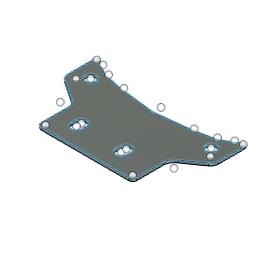
prop bracket (Autodesk Fusion 360 design; units mm, degrees)
Autodesk Fusion 360 part; units mm, degrees
sketch "sketch 344" plane through (0, 0, 1390) normal (0, 0, -1) x (1, 0, 0)
  circle A0 centre (6470.3364, 391.9726) radius 6.75
  circle A1 centre (6317.9364, 391.9726) radius 6.75
  line L0 (6410.85, 446.765) -> (6410.85, 453.115)
  arc A2 (6410.85, 453.115) -> (6424.35, 453.115) centre (6417.6, 453.115) cw
  line L1 (6424.35, 453.115) -> (6424.35, 446.765)
  arc A3 (6424.35, 446.765) -> (6410.85, 446.765) centre (6417.6, 446.765) cw
  line L2 (6367.75, 453.172) -> (6367.75, 446.828)
  arc A4 (6367.75, 446.828) -> (6354.25, 446.828) centre (6361, 446.828) cw
  line L3 (6354.25, 446.828) -> (6354.25, 453.172)
  arc A5 (6354.25, 453.172) -> (6367.75, 453.172) centre (6361, 453.172) cw
  line L4 (6455.7, 437.7) -> (6455.7, 471.6807)
  arc A6 (6455.7, 471.6807) -> (6450.62, 476.7607) centre (6450.62, 471.6807) ccw
  line L5 (6340.255, 476.7607) -> (6450.62, 476.7607)
  arc A7 (6340.255, 476.7607) -> (6335.175, 471.6807) centre (6340.255, 471.6807) ccw
  line L6 (6335.175, 437.7001) -> (6335.175, 471.6807)
  arc A8 (6330.4473, 428.3006) -> (6335.175, 437.7001) centre (6324.513, 437.1741) ccw
  line L7 (6303.3983, 410.211) -> (6330.4473, 428.3006)
  arc A9 (6303.3983, 410.211) -> (6298.8864, 401.7656) centre (6309.0464, 401.7656) ccw
  line L8 (6298.8864, 401.7656) -> (6298.8864, 367.9042)
  arc A10 (6298.8864, 367.9042) -> (6303.0986, 365.9924) centre (6301.4264, 367.9042) ccw
  line L9 (6309.1204, 371.2594) -> (6303.0986, 365.9924)
  arc A11 (6309.6287, 371.6052) -> (6309.1204, 371.2594) centre (6310.7926, 369.3475) ccw
  line L10 (6323.9162, 378.9712) -> (6309.6287, 371.6052)
  arc A12 (6324.5666, 379.2011) -> (6323.9162, 378.9712) centre (6325.0801, 376.7135) ccw
  line L11 (6349.1728, 384.2811) -> (6324.5666, 379.2011)
  arc A13 (6349.398, 384.3171) -> (6349.1728, 384.2811) centre (6349.6864, 381.7935) ccw
  line L12 (6349.398, 384.3171) -> (6392.9828, 389.2982)
  arc A14 (6395.29, 389.2982) -> (6392.9828, 389.2982) centre (6394.1364, 379.2039) ccw
  line L13 (6395.29, 389.2982) -> (6438.8748, 384.3171)
  arc A15 (6439.0999, 384.2811) -> (6438.8748, 384.3171) centre (6438.5864, 381.7935) ccw
  line L14 (6439.0999, 384.2811) -> (6463.7062, 379.2011)
  arc A16 (6464.3565, 378.9712) -> (6463.7062, 379.2011) centre (6463.1926, 376.7135) ccw
  line L15 (6464.3565, 378.9712) -> (6478.644, 371.6054)
  arc A17 (6479.1524, 371.2596) -> (6478.644, 371.6054) centre (6477.4801, 369.3477) ccw
  line L16 (6479.1524, 371.2596) -> (6485.1741, 365.9925)
  arc A18 (6485.1741, 365.9925) -> (6489.3864, 367.9043) centre (6486.8464, 367.9043) ccw
  line L17 (6489.3864, 401.9194) -> (6489.3864, 367.9043)
  arc A19 (6489.3864, 401.9194) -> (6485.0731, 410.2286) centre (6479.2264, 401.9194) ccw
  line L18 (6462.2651, 426.2773) -> (6485.0731, 410.2286)
  arc A20 (6455.7, 437.7) -> (6462.2651, 426.2773) centre (6468.9198, 437.7) ccw
extrude "Extrude1" add sketch "sketch 344" along normal blind 3.175
